Autodesk Inventor part; units mm, degrees
(part 2 of 2)
sketch "Sketch18" plane through (0, 0, -25.4) normal (0, 0, -1) x (-1, 0, 0)
  line L0 (16.4928, 228.3099) -> (15.5678, 226.2451) projected
  line L1 (15.5678, 226.2451) -> (12.4738, 226.4368) projected
  line L2 (12.4738, 226.4368) -> (11.8107, 228.5999) projected
  arc A0 (11.8107, 228.5999) -> (-2.4172, 228.892) centre (0, 0) ccw projected
  line L3 (-2.4172, 228.892) -> (-3.1685, 226.758) projected
  line L4 (-3.1685, 226.758) -> (-6.2678, 226.6935) projected
  line L5 (-6.2678, 226.6935) -> (-7.1073, 228.7944) projected
  arc A1 (-7.1073, 228.7944) -> (-11.8741, 228.5966) centre (0, 0) ccw projected
  line L6 (-11.8741, 228.5966) -> (-12.5366, 226.4333) projected
  line L7 (-12.5366, 226.4333) -> (-15.6306, 226.2408) projected
  line L8 (-15.6306, 226.2408) -> (-16.5561, 228.3053) projected
  arc A2 (-16.5561, 228.3053) -> (-21.3107, 227.9106) centre (0, 0) ccw projected
  line L9 (-21.3107, 227.9106) -> (-21.8832, 225.7218) projected
  line L10 (-21.8832, 225.7218) -> (-24.9666, 225.4016) projected
  line L11 (-24.9666, 225.4016) -> (-25.9767, 227.4261) projected
  arc A3 (-25.9767, 227.4261) -> (-30.7109, 226.8353) centre (0, 0) ccw projected
  line L12 (-30.7109, 226.8353) -> (-31.1925, 224.6247) projected
  line L13 (-31.1925, 224.6247) -> (-34.26, 224.1773) projected
  line L14 (-34.26, 224.1773) -> (-35.3529, 226.1583) projected
  arc A4 (-35.3529, 226.1583) -> (-40.0586, 225.3724) centre (0, 0) ccw projected
  line L15 (-40.0586, 225.3724) -> (-40.4484, 223.1438) projected
  line L16 (-40.4484, 223.1438) -> (-43.4949, 222.57) projected
  line L17 (-43.4949, 222.57) -> (-44.6687, 224.5042) projected
  arc A5 (-44.6687, 224.5042) -> (-49.3379, 223.5244) centre (0, 0) ccw projected
  line L18 (-49.3379, 223.5244) -> (-49.6353, 221.2816) projected
  line L19 (-49.6353, 221.2816) -> (-52.6554, 220.5825) projected
  line L20 (-52.6554, 220.5825) -> (-53.9082, 222.4664) projected
  arc A6 (-53.9082, 222.4664) -> (-58.5329, 221.2946) centre (0, 0) ccw projected
  line L21 (-58.5329, 221.2946) -> (-58.7374, 219.0414) projected
  line L22 (-58.7374, 219.0414) -> (-61.726, 218.218) projected
  line L23 (-61.726, 218.218) -> (-63.0555, 220.0486) projected
  arc A7 (-63.0555, 220.0486) -> (-67.6279, 218.6867) centre (0, 0) ccw projected
  line L24 (-67.6279, 218.6867) -> (-67.7391, 216.427) projected
  line L25 (-67.7391, 216.427) -> (-70.6911, 215.4808) projected
  line L26 (-70.6911, 215.4808) -> (-72.0952, 217.2549) projected
  arc A8 (-72.0952, 217.2549) -> (-76.6074, 215.7052) centre (0, 0) ccw projected
  line L27 (-76.6074, 215.7052) -> (-76.625, 213.4428) projected
  line L28 (-76.625, 213.4428) -> (-79.5355, 212.3754) projected
  line L29 (-79.5355, 212.3754) -> (-81.0116, 214.09) projected
  arc A9 (-81.0116, 214.09) -> (-85.4559, 212.3551) centre (0, 0) ccw projected
  line L30 (-85.4559, 212.3551) -> (-85.3801, 210.0939) projected
  line L31 (-85.3801, 210.0939) -> (-88.244, 208.9072) projected
  line L32 (-88.244, 208.9072) -> (-89.7897, 210.5593) projected
  arc A10 (-89.7897, 210.5593) -> (-94.1585, 208.6422) centre (0, 0) ccw projected
  line L33 (-94.1585, 208.6422) -> (-93.9893, 206.3861) projected
  line L34 (-93.9893, 206.3861) -> (-96.8017, 205.0821) projected
  line L35 (-96.8017, 205.0821) -> (-98.4143, 206.6689) projected
  arc A11 (-98.4143, 206.6689) -> (-102.7002, 204.5729) centre (0, 0) ccw projected
  line L36 (-102.7002, 204.5729) -> (-102.4379, 202.3257) projected
  line L37 (-102.4379, 202.3257) -> (-105.194, 200.9065) projected
  line L38 (-105.194, 200.9065) -> (-106.8709, 202.4254) projected
  arc A12 (-106.8709, 202.4254) -> (-111.0664, 200.1541) centre (0, 0) ccw projected
  line L39 (-111.0664, 200.1541) -> (-110.7115, 197.9196) projected
  line L40 (-110.7115, 197.9196) -> (-113.4066, 196.3878) projected
  line L41 (-113.4066, 196.3878) -> (-115.1448, 197.836) projected
  arc A13 (-115.1448, 197.836) -> (-119.2429, 195.3933) centre (0, 0) ccw projected
  line L42 (-119.2429, 195.3933) -> (-118.7959, 193.1754) projected
  line L43 (-118.7959, 193.1754) -> (-121.4254, 191.5335) projected
  line L44 (-121.4254, 191.5335) -> (-123.222, 192.9086) projected
  arc A14 (-123.222, 192.9086) -> (-127.2157, 190.2987) centre (0, 0) ccw projected
  line L45 (-127.2157, 190.2987) -> (-126.6774, 188.1011) projected
  line L46 (-126.6774, 188.1011) -> (-129.2368, 186.352) projected
  line L47 (-129.2368, 186.352) -> (-131.0887, 187.6517) projected
  arc A15 (-131.0887, 187.6517) -> (-134.9711, 184.8789) centre (0, 0) ccw projected
  line L48 (-134.9711, 184.8789) -> (-134.3425, 182.7055) projected
  line L49 (-134.3425, 182.7055) -> (-136.8274, 180.8521) projected
  line L50 (-136.8274, 180.8521) -> (-138.7314, 182.0742) projected
  arc A16 (-138.7314, 182.0742) -> (-142.4959, 179.1433) centre (0, 0) ccw projected
  line L51 (-142.4959, 179.1433) -> (-141.778, 176.9977) projected
  line L52 (-141.778, 176.9977) -> (-144.1842, 175.0432) projected
  line L53 (-144.1842, 175.0432) -> (-146.1371, 176.1856) projected
  arc A17 (-146.1371, 176.1856) -> (-149.7773, 173.1016) centre (0, 0) ccw projected
  line L54 (-149.7773, 173.1016) -> (-148.9713, 170.9876) projected
  line L55 (-148.9713, 170.9876) -> (-151.2947, 168.9353) projected
  line L56 (-151.2947, 168.9353) -> (-153.2931, 169.9959) projected
  arc A18 (-153.2931, 169.9959) -> (-156.8028, 166.7642) centre (0, 0) ccw projected
  line L57 (-156.8028, 166.7642) -> (-155.9101, 164.6853) projected
  line L58 (-155.9101, 164.6853) -> (-158.1467, 162.5387) projected
  line L59 (-158.1467, 162.5387) -> (-160.1873, 163.5159) projected
  arc A19 (-160.1873, 163.5159) -> (-163.5603, 160.1419) centre (0, 0) ccw projected
  line L60 (-163.5603, 160.1419) -> (-162.5826, 158.1016) projected
  line L61 (-162.5826, 158.1016) -> (-164.7285, 155.8644) projected
  line L62 (-164.7285, 155.8644) -> (-166.8077, 156.7565) projected
  arc A20 (-166.8077, 156.7565) -> (-170.0385, 153.246) centre (0, 0) ccw projected
  line L63 (-170.0385, 153.246) -> (-168.9772, 151.2478) projected
  line L64 (-168.9772, 151.2478) -> (-171.0289, 148.9239) projected
  line L65 (-171.0289, 148.9239) -> (-173.1432, 149.7292) projected
  arc A21 (-173.1432, 149.7292) -> (-176.2261, 146.0882) centre (0, 0) ccw projected
  line L66 (-176.2261, 146.0882) -> (-175.0832, 144.1357) projected
  line L67 (-175.0832, 144.1357) -> (-177.0371, 141.7289) projected
  line L68 (-177.0371, 141.7289) -> (-179.1828, 142.4462) projected
  arc A22 (-179.1828, 142.4462) -> (-182.1127, 138.6809) centre (0, 0) ccw projected
  line L69 (-182.1127, 138.6809) -> (-180.89, 136.7772) projected
  line L70 (-180.89, 136.7772) -> (-182.7428, 134.2918) projected
  line L71 (-182.7428, 134.2918) -> (-184.9163, 134.9198) projected
  arc A23 (-184.9163, 134.9198) -> (-187.6881, 131.0366) centre (0, 0) ccw projected
  line L72 (-187.6881, 131.0366) -> (-186.3878, 129.1851) projected
  line L73 (-186.3878, 129.1851) -> (-188.1363, 126.6252) projected
  line L74 (-188.1363, 126.6252) -> (-190.3339, 127.1629) projected
  arc A24 (-190.3339, 127.1629) -> (-192.9428, 123.1685) centre (0, 0) ccw projected
  line L75 (-192.9428, 123.1685) -> (-191.5672, 121.3723) projected
  line L76 (-191.5672, 121.3723) -> (-193.2084, 118.7423) projected
  line L77 (-193.2084, 118.7423) -> (-195.4264, 119.1887) projected
  arc A25 (-195.4264, 119.1887) -> (-197.8679, 115.0899) centre (0, 0) ccw projected
  line L78 (-197.8679, 115.0899) -> (-196.4192, 113.3521) projected
  line L79 (-196.4192, 113.3521) -> (-197.9503, 110.6566) projected
  line L80 (-197.9503, 110.6566) -> (-200.1849, 111.0109) projected
  arc A26 (-200.1849, 111.0109) -> (-202.455, 106.8147) centre (0, 0) ccw projected
  line L81 (-202.455, 106.8147) -> (-200.9357, 105.1382) projected
  line L82 (-200.9357, 105.1382) -> (-202.3541, 102.3818) projected
  line L83 (-202.3541, 102.3818) -> (-204.6014, 102.6434) projected
  arc A27 (-204.6014, 102.6434) -> (-206.6962, 98.357) centre (0, 0) ccw projected
  line L84 (-206.6962, 98.357) -> (-205.1089, 96.7448) projected
  line L85 (-205.1089, 96.7448) -> (-206.4122, 93.932) projected
  line L86 (-206.4122, 93.932) -> (-208.6684, 94.1006) projected
  arc A28 (-208.6684, 94.1006) -> (-210.5842, 89.7313) centre (0, 0) ccw projected
  line L87 (-210.5842, 89.7313) -> (-208.9317, 88.186) projected
  line L88 (-208.9317, 88.186) -> (-210.1176, 85.3218) projected
  line L89 (-210.1176, 85.3218) -> (-212.3788, 85.397) projected
  arc A29 (-212.3788, 85.397) -> (-214.1125, 80.9522) centre (0, 0) ccw projected
  line L90 (-214.1125, 80.9522) -> (-212.3975, 79.4766) projected
  line L91 (-212.3975, 79.4766) -> (-213.464, 76.5658) projected
  line L92 (-213.464, 76.5658) -> (-215.7264, 76.5475) projected
  arc A30 (-215.7264, 76.5475) -> (-217.2749, 72.0349) centre (0, 0) ccw projected
  line L93 (-217.2749, 72.0349) -> (-215.5004, 70.6313) projected
  line L94 (-215.5004, 70.6313) -> (-216.4458, 67.679) projected
  line L95 (-216.4458, 67.679) -> (-218.7055, 67.5672) projected
  arc A31 (-218.7055, 67.5672) -> (-220.0661, 62.9945) centre (0, 0) ccw projected
  line L96 (-220.0661, 62.9945) -> (-218.2352, 61.6655) projected
  line L97 (-218.2352, 61.6655) -> (-219.0577, 58.6766) projected
  line L98 (-219.0577, 58.6766) -> (-221.3108, 58.4715) projected
  arc A32 (-221.3108, 58.4715) -> (-222.4814, 53.8464) centre (0, 0) ccw projected
  line L99 (-222.4814, 53.8464) -> (-220.5971, 52.5942) projected
  line L100 (-220.5971, 52.5942) -> (-221.2954, 49.5739) projected
  line L101 (-221.2954, 49.5739) -> (-223.5381, 49.2759) projected
  arc A33 (-223.5381, 49.2759) -> (-224.5165, 44.6064) centre (0, 0) ccw projected
  line L102 (-224.5165, 44.6064) -> (-222.5821, 43.4331) projected
  line L103 (-222.5821, 43.4331) -> (-223.155, 40.3865) projected
  line L104 (-223.155, 40.3865) -> (-225.3835, 39.9961) projected
  arc A34 (-225.3835, 39.9961) -> (-226.1681, 35.2902) centre (0, 0) ccw projected
  line L105 (-226.1681, 35.2902) -> (-224.1868, 34.1978) projected
  line L106 (-224.1868, 34.1978) -> (-224.6333, 31.1302) projected
  line L107 (-224.6333, 31.1302) -> (-226.8438, 30.648) projected
  arc A35 (-226.8438, 30.648) -> (-227.4333, 25.9136) centre (0, 0) ccw projected
  line L108 (-227.4333, 25.9136) -> (-225.4085, 24.9041) projected
  line L109 (-225.4085, 24.9041) -> (-225.7279, 21.8206) projected
  line L110 (-225.7279, 21.8206) -> (-227.9165, 21.2475) projected
  arc A36 (-227.9165, 21.2475) -> (-228.3099, 16.4928) centre (0, 0) ccw projected
  line L111 (-228.3099, 16.4928) -> (-226.2451, 15.5678) projected
  line L112 (-226.2451, 15.5678) -> (-226.4368, 12.4738) projected
  line L113 (-226.4368, 12.4738) -> (-228.5999, 11.8107) projected
  arc A37 (-228.5999, 11.8107) -> (-228.7964, 7.0438) centre (0, 0) ccw projected
  line L114 (-228.7964, 7.0438) -> (-226.6952, 6.205) projected
  line L115 (-226.6952, 6.205) -> (-226.7588, 3.1056) projected
  line L116 (-226.7588, 3.1056) -> (-228.8927, 2.3537) projected
  arc A38 (-228.8927, 2.3537) -> (-228.892, -2.4172) centre (0, 0) ccw projected
  line L117 (-228.892, -2.4172) -> (-226.758, -3.1685) projected
  line L118 (-226.758, -3.1685) -> (-226.6935, -6.2678) projected
  line L119 (-226.6935, -6.2678) -> (-228.7944, -7.1073) projected
  arc A39 (-228.7944, -7.1073) -> (-228.5966, -11.8741) centre (0, 0) ccw projected
  line L120 (-228.5966, -11.8741) -> (-226.4333, -12.5366) projected
  line L121 (-226.4333, -12.5366) -> (-226.2408, -15.6306) projected
  line L122 (-226.2408, -15.6306) -> (-228.3053, -16.5561) projected
  arc A40 (-228.3053, -16.5561) -> (-227.9106, -21.3107) centre (0, 0) ccw projected
  line L123 (-227.9106, -21.3107) -> (-225.7218, -21.8832) projected
  line L124 (-225.7218, -21.8832) -> (-225.4016, -24.9666) projected
  line L125 (-225.4016, -24.9666) -> (-227.4261, -25.9767) projected
  arc A41 (-227.4261, -25.9767) -> (-226.8353, -30.7109) centre (0, 0) ccw projected
  line L126 (-226.8353, -30.7109) -> (-224.6247, -31.1925) projected
  line L127 (-224.6247, -31.1925) -> (-224.1773, -34.26) projected
  line L128 (-224.1773, -34.26) -> (-226.1583, -35.3529) projected
  arc A42 (-226.1583, -35.3529) -> (-225.3724, -40.0586) centre (0, 0) ccw projected
  line L129 (-225.3724, -40.0586) -> (-223.1438, -40.4484) projected
  line L130 (-223.1438, -40.4484) -> (-222.57, -43.4949) projected
  line L131 (-222.57, -43.4949) -> (-224.5042, -44.6687) projected
  arc A43 (-224.5042, -44.6687) -> (-223.5244, -49.3379) centre (0, 0) ccw projected
  line L132 (-223.5244, -49.3379) -> (-221.2816, -49.6353) projected
  line L133 (-221.2816, -49.6353) -> (-220.5825, -52.6554) projected
  line L134 (-220.5825, -52.6554) -> (-222.4664, -53.9082) projected
  arc A44 (-222.4664, -53.9082) -> (-221.2946, -58.5329) centre (0, 0) ccw projected
  line L135 (-221.2946, -58.5329) -> (-219.0414, -58.7374) projected
  line L136 (-219.0414, -58.7374) -> (-218.218, -61.726) projected
  line L137 (-218.218, -61.726) -> (-220.0486, -63.0555) projected
  arc A45 (-220.0486, -63.0555) -> (-218.6867, -67.6279) centre (0, 0) ccw projected
  line L138 (-218.6867, -67.6279) -> (-216.427, -67.7391) projected
  line L139 (-216.427, -67.7391) -> (-215.4808, -70.6911) projected
  line L140 (-215.4808, -70.6911) -> (-217.2549, -72.0952) projected
  arc A46 (-217.2549, -72.0952) -> (-215.7052, -76.6074) centre (0, 0) ccw projected
  line L141 (-215.7052, -76.6074) -> (-213.4428, -76.625) projected
  line L142 (-213.4428, -76.625) -> (-212.3754, -79.5355) projected
  line L143 (-212.3754, -79.5355) -> (-214.09, -81.0116) projected
  arc A47 (-214.09, -81.0116) -> (-212.3551, -85.4559) centre (0, 0) ccw projected
  line L144 (-212.3551, -85.4559) -> (-210.0939, -85.3801) projected
  line L145 (-210.0939, -85.3801) -> (-208.9072, -88.244) projected
  line L146 (-208.9072, -88.244) -> (-210.5593, -89.7897) projected
  arc A48 (-210.5593, -89.7897) -> (-208.6422, -94.1585) centre (0, 0) ccw projected
  line L147 (-208.6422, -94.1585) -> (-206.3861, -93.9893) projected
  line L148 (-206.3861, -93.9893) -> (-205.0821, -96.8017) projected
  line L149 (-205.0821, -96.8017) -> (-206.6689, -98.4143) projected
  arc A49 (-206.6689, -98.4143) -> (-204.5729, -102.7002) centre (0, 0) ccw projected
  line L150 (-204.5729, -102.7002) -> (-202.3257, -102.4379) projected
  line L151 (-202.3257, -102.4379) -> (-200.9065, -105.194) projected
  line L152 (-200.9065, -105.194) -> (-202.4254, -106.8709) projected
  arc A50 (-202.4254, -106.8709) -> (-200.1541, -111.0664) centre (0, 0) ccw projected
  line L153 (-200.1541, -111.0664) -> (-197.9196, -110.7115) projected
  line L154 (-197.9196, -110.7115) -> (-196.3878, -113.4066) projected
  line L155 (-196.3878, -113.4066) -> (-197.836, -115.1448) projected
  arc A51 (-197.836, -115.1448) -> (-195.3933, -119.2429) centre (0, 0) ccw projected
  line L156 (-195.3933, -119.2429) -> (-193.1754, -118.7959) projected
  line L157 (-193.1754, -118.7959) -> (-191.5335, -121.4254) projected
  line L158 (-191.5335, -121.4254) -> (-192.9086, -123.222) projected
  arc A52 (-192.9086, -123.222) -> (-190.2987, -127.2157) centre (0, 0) ccw projected
  line L159 (-190.2987, -127.2157) -> (-188.1011, -126.6774) projected
  line L160 (-188.1011, -126.6774) -> (-186.352, -129.2368) projected
  line L161 (-186.352, -129.2368) -> (-187.6517, -131.0887) projected
  arc A53 (-187.6517, -131.0887) -> (-184.8789, -134.9711) centre (0, 0) ccw projected
  line L162 (-184.8789, -134.9711) -> (-182.7055, -134.3425) projected
  line L163 (-182.7055, -134.3425) -> (-180.8521, -136.8274) projected
  line L164 (-180.8521, -136.8274) -> (-182.0742, -138.7314) projected
  arc A54 (-182.0742, -138.7314) -> (-179.1433, -142.4959) centre (0, 0) ccw projected
  line L165 (-179.1433, -142.4959) -> (-176.9977, -141.778) projected
  line L166 (-176.9977, -141.778) -> (-175.0432, -144.1842) projected
  line L167 (-175.0432, -144.1842) -> (-176.1856, -146.1371) projected
  arc A55 (-176.1856, -146.1371) -> (-173.1016, -149.7773) centre (0, 0) ccw projected
  line L168 (-173.1016, -149.7773) -> (-170.9876, -148.9713) projected
  line L169 (-170.9876, -148.9713) -> (-168.9353, -151.2947) projected
  line L170 (-168.9353, -151.2947) -> (-169.9959, -153.2931) projected
  arc A56 (-169.9959, -153.2931) -> (-166.7642, -156.8028) centre (0, 0) ccw projected
  line L171 (-166.7642, -156.8028) -> (-164.6853, -155.9101) projected
  line L172 (-164.6853, -155.9101) -> (-162.5387, -158.1467) projected
  line L173 (-162.5387, -158.1467) -> (-163.5159, -160.1873) projected
  arc A57 (-163.5159, -160.1873) -> (-160.1419, -163.5603) centre (0, 0) ccw projected
  line L174 (-160.1419, -163.5603) -> (-158.1016, -162.5826) projected
  line L175 (-158.1016, -162.5826) -> (-155.8644, -164.7285) projected
  line L176 (-155.8644, -164.7285) -> (-156.7565, -166.8077) projected
  arc A58 (-156.7565, -166.8077) -> (-153.246, -170.0385) centre (0, 0) ccw projected
  line L177 (-153.246, -170.0385) -> (-151.2478, -168.9772) projected
  line L178 (-151.2478, -168.9772) -> (-148.9239, -171.0289) projected
  line L179 (-148.9239, -171.0289) -> (-149.7292, -173.1432) projected
  arc A59 (-149.7292, -173.1432) -> (-146.0882, -176.2261) centre (0, 0) ccw projected
  line L180 (-146.0882, -176.2261) -> (-144.1357, -175.0832) projected
  line L181 (-144.1357, -175.0832) -> (-141.7289, -177.0371) projected
  line L182 (-141.7289, -177.0371) -> (-142.4462, -179.1828) projected
  arc A60 (-142.4462, -179.1828) -> (-138.6809, -182.1127) centre (0, 0) ccw projected
  line L183 (-138.6809, -182.1127) -> (-136.7772, -180.89) projected
  line L184 (-136.7772, -180.89) -> (-134.2918, -182.7428) projected
  line L185 (-134.2918, -182.7428) -> (-134.9198, -184.9163) projected
  arc A61 (-134.9198, -184.9163) -> (-131.0366, -187.6881) centre (0, 0) ccw projected
  line L186 (-131.0366, -187.6881) -> (-129.1851, -186.3878) projected
  line L187 (-129.1851, -186.3878) -> (-126.6252, -188.1363) projected
  line L188 (-126.6252, -188.1363) -> (-127.1629, -190.3339) projected
  arc A62 (-127.1629, -190.3339) -> (-123.1685, -192.9428) centre (0, 0) ccw projected
  line L189 (-123.1685, -192.9428) -> (-121.3723, -191.5672) projected
  line L190 (-121.3723, -191.5672) -> (-118.7423, -193.2084) projected
  line L191 (-118.7423, -193.2084) -> (-119.1887, -195.4264) projected
  arc A63 (-119.1887, -195.4264) -> (-115.0899, -197.8679) centre (0, 0) ccw projected
  line L192 (-115.0899, -197.8679) -> (-113.3521, -196.4192) projected
  line L193 (-113.3521, -196.4192) -> (-110.6566, -197.9503) projected
  line L194 (-110.6566, -197.9503) -> (-111.0109, -200.1849) projected
  arc A64 (-111.0109, -200.1849) -> (-106.8147, -202.455) centre (0, 0) ccw projected
  line L195 (-106.8147, -202.455) -> (-105.1382, -200.9357) projected
  line L196 (-105.1382, -200.9357) -> (-102.3818, -202.3541) projected
  line L197 (-102.3818, -202.3541) -> (-102.6434, -204.6014) projected
  arc A65 (-102.6434, -204.6014) -> (-98.357, -206.6962) centre (0, 0) ccw projected
  line L198 (-98.357, -206.6962) -> (-96.7448, -205.1089) projected
  line L199 (-96.7448, -205.1089) -> (-93.932, -206.4122) projected
  line L200 (-93.932, -206.4122) -> (-94.1006, -208.6684) projected
  arc A66 (-94.1006, -208.6684) -> (-89.7313, -210.5842) centre (0, 0) ccw projected
  line L201 (-89.7313, -210.5842) -> (-88.186, -208.9317) projected
  line L202 (-88.186, -208.9317) -> (-85.3218, -210.1176) projected
  line L203 (-85.3218, -210.1176) -> (-85.397, -212.3788) projected
  arc A67 (-85.397, -212.3788) -> (-80.9522, -214.1125) centre (0, 0) ccw projected
  line L204 (-80.9522, -214.1125) -> (-79.4766, -212.3975) projected
  line L205 (-79.4766, -212.3975) -> (-76.5658, -213.464) projected
  line L206 (-76.5658, -213.464) -> (-76.5475, -215.7264) projected
  arc A68 (-76.5475, -215.7264) -> (-72.0349, -217.2749) centre (0, 0) ccw projected
  line L207 (-72.0349, -217.2749) -> (-70.6313, -215.5004) projected
  line L208 (-70.6313, -215.5004) -> (-67.679, -216.4458) projected
  line L209 (-67.679, -216.4458) -> (-67.5672, -218.7055) projected
  arc A69 (-67.5672, -218.7055) -> (-62.9945, -220.0661) centre (0, 0) ccw projected
  line L210 (-62.9945, -220.0661) -> (-61.6655, -218.2352) projected
  line L211 (-61.6655, -218.2352) -> (-58.6766, -219.0577) projected
  line L212 (-58.6766, -219.0577) -> (-58.4715, -221.3108) projected
  arc A70 (-58.4715, -221.3108) -> (-53.8464, -222.4814) centre (0, 0) ccw projected
  line L213 (-53.8464, -222.4814) -> (-52.5942, -220.5971) projected
  line L214 (-52.5942, -220.5971) -> (-49.5739, -221.2954) projected
  line L215 (-49.5739, -221.2954) -> (-49.2759, -223.5381) projected
  arc A71 (-49.2759, -223.5381) -> (-44.6064, -224.5165) centre (0, 0) ccw projected
  line L216 (-44.6064, -224.5165) -> (-43.4331, -222.5821) projected
  line L217 (-43.4331, -222.5821) -> (-40.3865, -223.155) projected
  line L218 (-40.3865, -223.155) -> (-39.9961, -225.3835) projected
  arc A72 (-39.9961, -225.3835) -> (-35.2902, -226.1681) centre (0, 0) ccw projected
  line L219 (-35.2902, -226.1681) -> (-34.1978, -224.1868) projected
  line L220 (-34.1978, -224.1868) -> (-31.1302, -224.6333) projected
  line L221 (-31.1302, -224.6333) -> (-30.648, -226.8438) projected
  arc A73 (-30.648, -226.8438) -> (-25.9136, -227.4333) centre (0, 0) ccw projected
  line L222 (-25.9136, -227.4333) -> (-24.9041, -225.4085) projected
  line L223 (-24.9041, -225.4085) -> (-21.8206, -225.7279) projected
  line L224 (-21.8206, -225.7279) -> (-21.2475, -227.9165) projected
  arc A74 (-21.2475, -227.9165) -> (-16.4928, -228.3099) centre (0, 0) ccw projected
  line L225 (-16.4928, -228.3099) -> (-15.5678, -226.2451) projected
  line L226 (-15.5678, -226.2451) -> (-12.4738, -226.4368) projected
  line L227 (-12.4738, -226.4368) -> (-11.8107, -228.5999) projected
  arc A75 (-11.8107, -228.5999) -> (-7.0438, -228.7964) centre (0, 0) ccw projected
  line L228 (-7.0438, -228.7964) -> (-6.205, -226.6952) projected
  line L229 (-6.205, -226.6952) -> (-3.1056, -226.7588) projected
  line L230 (-3.1056, -226.7588) -> (-2.3537, -228.8927) projected
  arc A76 (-2.3537, -228.8927) -> (2.4172, -228.892) centre (0, 0) ccw projected
  line L231 (2.4172, -228.892) -> (3.1685, -226.758) projected
  line L232 (3.1685, -226.758) -> (6.2678, -226.6935) projected
  line L233 (6.2678, -226.6935) -> (7.1073, -228.7944) projected
  arc A77 (7.1073, -228.7944) -> (11.8741, -228.5966) centre (0, 0) ccw projected
  line L234 (11.8741, -228.5966) -> (12.5366, -226.4333) projected
  line L235 (12.5366, -226.4333) -> (15.6306, -226.2408) projected
  line L236 (15.6306, -226.2408) -> (16.5561, -228.3053) projected
  arc A78 (16.5561, -228.3053) -> (21.3107, -227.9106) centre (0, 0) ccw projected
  line L237 (21.3107, -227.9106) -> (21.8832, -225.7218) projected
  line L238 (21.8832, -225.7218) -> (24.9666, -225.4016) projected
  line L239 (24.9666, -225.4016) -> (25.9767, -227.4261) projected
  arc A79 (25.9767, -227.4261) -> (30.7109, -226.8353) centre (0, 0) ccw projected
  line L240 (30.7109, -226.8353) -> (31.1925, -224.6247) projected
  line L241 (31.1925, -224.6247) -> (34.26, -224.1773) projected
  line L242 (34.26, -224.1773) -> (35.3529, -226.1583) projected
  arc A80 (35.3529, -226.1583) -> (40.0586, -225.3724) centre (0, 0) ccw projected
  line L243 (40.0586, -225.3724) -> (40.4484, -223.1438) projected
  line L244 (40.4484, -223.1438) -> (43.4949, -222.57) projected
  line L245 (43.4949, -222.57) -> (44.6687, -224.5042) projected
  arc A81 (44.6687, -224.5042) -> (49.3379, -223.5244) centre (0, 0) ccw projected
  line L246 (49.3379, -223.5244) -> (49.6353, -221.2816) projected
  line L247 (49.6353, -221.2816) -> (52.6554, -220.5825) projected
  line L248 (52.6554, -220.5825) -> (53.9082, -222.4664) projected
  arc A82 (53.9082, -222.4664) -> (58.5329, -221.2946) centre (0, 0) ccw projected
  line L249 (58.5329, -221.2946) -> (58.7374, -219.0414) projected
  line L250 (58.7374, -219.0414) -> (61.726, -218.218) projected
  line L251 (61.726, -218.218) -> (63.0555, -220.0486) projected
  arc A83 (63.0555, -220.0486) -> (67.6279, -218.6867) centre (0, 0) ccw projected
  line L252 (67.6279, -218.6867) -> (67.7391, -216.427) projected
  line L253 (67.7391, -216.427) -> (70.6911, -215.4808) projected
  line L254 (70.6911, -215.4808) -> (72.0952, -217.2549) projected
  arc A84 (72.0952, -217.2549) -> (76.6074, -215.7052) centre (0, 0) ccw projected
  line L255 (76.6074, -215.7052) -> (76.625, -213.4428) projected
  line L256 (76.625, -213.4428) -> (79.5355, -212.3754) projected
  line L257 (79.5355, -212.3754) -> (81.0116, -214.09) projected
  arc A85 (81.0116, -214.09) -> (85.4559, -212.3551) centre (0, 0) ccw projected
  line L258 (85.4559, -212.3551) -> (85.3801, -210.0939) projected
  line L259 (85.3801, -210.0939) -> (88.244, -208.9072) projected
  line L260 (88.244, -208.9072) -> (89.7897, -210.5593) projected
  arc A86 (89.7897, -210.5593) -> (94.1585, -208.6422) centre (0, 0) ccw projected
  line L261 (94.1585, -208.6422) -> (93.9893, -206.3861) projected
  line L262 (93.9893, -206.3861) -> (96.8017, -205.0821) projected
  line L263 (96.8017, -205.0821) -> (98.4143, -206.6689) projected
  arc A87 (98.4143, -206.6689) -> (102.7002, -204.5729) centre (0, 0) ccw projected
  line L264 (102.7002, -204.5729) -> (102.4379, -202.3257) projected
  line L265 (102.4379, -202.3257) -> (105.194, -200.9065) projected
  line L266 (105.194, -200.9065) -> (106.8709, -202.4254) projected
  arc A88 (106.8709, -202.4254) -> (111.0664, -200.1541) centre (0, 0) ccw projected
  line L267 (111.0664, -200.1541) -> (110.7115, -197.9196) projected
  line L268 (110.7115, -197.9196) -> (113.4066, -196.3878) projected
  line L269 (113.4066, -196.3878) -> (115.1448, -197.836) projected
  arc A89 (115.1448, -197.836) -> (119.2429, -195.3933) centre (0, 0) ccw projected
  line L270 (119.2429, -195.3933) -> (118.7959, -193.1754) projected
  line L271 (118.7959, -193.1754) -> (121.4254, -191.5335) projected
  line L272 (121.4254, -191.5335) -> (123.222, -192.9086) projected
  arc A90 (123.222, -192.9086) -> (127.2157, -190.2987) centre (0, 0) ccw projected
  line L273 (127.2157, -190.2987) -> (126.6774, -188.1011) projected
  line L274 (126.6774, -188.1011) -> (129.2368, -186.352) projected
  line L275 (129.2368, -186.352) -> (131.0887, -187.6517) projected
  arc A91 (131.0887, -187.6517) -> (134.9711, -184.8789) centre (0, 0) ccw projected
  line L276 (134.9711, -184.8789) -> (134.3425, -182.7055) projected
  line L277 (134.3425, -182.7055) -> (136.8274, -180.8521) projected
  line L278 (136.8274, -180.8521) -> (138.7314, -182.0742) projected
  arc A92 (138.7314, -182.0742) -> (142.4959, -179.1433) centre (0, 0) ccw projected
  line L279 (142.4959, -179.1433) -> (141.778, -176.9977) projected
  line L280 (141.778, -176.9977) -> (144.1842, -175.0432) projected
  line L281 (144.1842, -175.0432) -> (146.1371, -176.1856) projected
  arc A93 (146.1371, -176.1856) -> (149.7773, -173.1016) centre (0, 0) ccw projected
  line L282 (149.7773, -173.1016) -> (148.9713, -170.9876) projected
  line L283 (148.9713, -170.9876) -> (151.2947, -168.9353) projected
  line L284 (151.2947, -168.9353) -> (153.2931, -169.9959) projected
  arc A94 (153.2931, -169.9959) -> (156.8028, -166.7642) centre (0, 0) ccw projected
  line L285 (156.8028, -166.7642) -> (155.9101, -164.6853) projected
  line L286 (155.9101, -164.6853) -> (158.1467, -162.5387) projected
  line L287 (158.1467, -162.5387) -> (160.1873, -163.5159) projected
  arc A95 (160.1873, -163.5159) -> (163.5603, -160.1419) centre (0, 0) ccw projected
  line L288 (163.5603, -160.1419) -> (162.5826, -158.1016) projected
  line L289 (162.5826, -158.1016) -> (164.7285, -155.8644) projected
  line L290 (164.7285, -155.8644) -> (166.8077, -156.7565) projected
  arc A96 (166.8077, -156.7565) -> (170.0385, -153.246) centre (0, 0) ccw projected
  line L291 (170.0385, -153.246) -> (168.9772, -151.2478) projected
  line L292 (168.9772, -151.2478) -> (171.0289, -148.9239) projected
  line L293 (171.0289, -148.9239) -> (173.1432, -149.7292) projected
  arc A97 (173.1432, -149.7292) -> (176.2261, -146.0882) centre (0, 0) ccw projected
  line L294 (176.2261, -146.0882) -> (175.0832, -144.1357) projected
  line L295 (175.0832, -144.1357) -> (177.0371, -141.7289) projected
  line L296 (177.0371, -141.7289) -> (179.1828, -142.4462) projected
  arc A98 (179.1828, -142.4462) -> (182.1127, -138.6809) centre (0, 0) ccw projected
  line L297 (182.1127, -138.6809) -> (180.89, -136.7772) projected
  line L298 (180.89, -136.7772) -> (182.7428, -134.2918) projected
  line L299 (182.7428, -134.2918) -> (184.9163, -134.9198) projected
  arc A99 (184.9163, -134.9198) -> (187.6881, -131.0366) centre (0, 0) ccw projected
  line L300 (187.6881, -131.0366) -> (186.3878, -129.1851) projected
  line L301 (186.3878, -129.1851) -> (188.1363, -126.6252) projected
  line L302 (188.1363, -126.6252) -> (190.3339, -127.1629) projected
  arc A100 (190.3339, -127.1629) -> (192.9428, -123.1685) centre (0, 0) ccw projected
  line L303 (192.9428, -123.1685) -> (191.5672, -121.3723) projected
  line L304 (191.5672, -121.3723) -> (193.2084, -118.7423) projected
  line L305 (193.2084, -118.7423) -> (195.4264, -119.1887) projected
  arc A101 (195.4264, -119.1887) -> (197.8679, -115.0899) centre (0, 0) ccw projected
  line L306 (197.8679, -115.0899) -> (196.4192, -113.3521) projected
  line L307 (196.4192, -113.3521) -> (197.9503, -110.6566) projected
  line L308 (197.9503, -110.6566) -> (200.1849, -111.0109) projected
  arc A102 (200.1849, -111.0109) -> (202.455, -106.8147) centre (0, 0) ccw projected
  line L309 (202.455, -106.8147) -> (200.9357, -105.1382) projected
  line L310 (200.9357, -105.1382) -> (202.3541, -102.3818) projected
  line L311 (202.3541, -102.3818) -> (204.6014, -102.6434) projected
  arc A103 (204.6014, -102.6434) -> (206.6962, -98.357) centre (0, 0) ccw projected
  line L312 (206.6962, -98.357) -> (205.1089, -96.7448) projected
  line L313 (205.1089, -96.7448) -> (206.4122, -93.932) projected
  line L314 (206.4122, -93.932) -> (208.6684, -94.1006) projected
  arc A104 (208.6684, -94.1006) -> (210.5842, -89.7313) centre (0, 0) ccw projected
  line L315 (210.5842, -89.7313) -> (208.9317, -88.186) projected
  line L316 (208.9317, -88.186) -> (210.1176, -85.3218) projected
  line L317 (210.1176, -85.3218) -> (212.3788, -85.397) projected
  arc A105 (212.3788, -85.397) -> (214.1125, -80.9522) centre (0, 0) ccw projected
  line L318 (214.1125, -80.9522) -> (212.3975, -79.4766) projected
  line L319 (212.3975, -79.4766) -> (213.464, -76.5658) projected
  line L320 (213.464, -76.5658) -> (215.7264, -76.5475) projected
  arc A106 (215.7264, -76.5475) -> (217.2749, -72.0349) centre (0, 0) ccw projected
  line L321 (217.2749, -72.0349) -> (215.5004, -70.6313) projected
  line L322 (215.5004, -70.6313) -> (216.4458, -67.679) projected
  line L323 (216.4458, -67.679) -> (218.7055, -67.5672) projected
  arc A107 (218.7055, -67.5672) -> (220.0661, -62.9945) centre (0, 0) ccw projected
  line L324 (220.0661, -62.9945) -> (218.2352, -61.6655) projected
  line L325 (218.2352, -61.6655) -> (219.0577, -58.6766) projected
  line L326 (219.0577, -58.6766) -> (221.3108, -58.4715) projected
  arc A108 (221.3108, -58.4715) -> (222.4814, -53.8464) centre (0, 0) ccw projected
  line L327 (222.4814, -53.8464) -> (220.5971, -52.5942) projected
  line L328 (220.5971, -52.5942) -> (221.2954, -49.5739) projected
  line L329 (221.2954, -49.5739) -> (223.5381, -49.2759) projected
  arc A109 (223.5381, -49.2759) -> (224.5165, -44.6064) centre (0, 0) ccw projected
  line L330 (224.5165, -44.6064) -> (222.5821, -43.4331) projected
  line L331 (222.5821, -43.4331) -> (223.155, -40.3865) projected
  line L332 (223.155, -40.3865) -> (225.3835, -39.9961) projected
  arc A110 (225.3835, -39.9961) -> (226.1681, -35.2902) centre (0, 0) ccw projected
  line L333 (226.1681, -35.2902) -> (224.1868, -34.1978) projected
  line L334 (224.1868, -34.1978) -> (224.6333, -31.1302) projected
  line L335 (224.6333, -31.1302) -> (226.8438, -30.648) projected
  arc A111 (226.8438, -30.648) -> (227.4333, -25.9136) centre (0, 0) ccw projected
  line L336 (227.4333, -25.9136) -> (225.4085, -24.9041) projected
  line L337 (225.4085, -24.9041) -> (225.7279, -21.8206) projected
  line L338 (225.7279, -21.8206) -> (227.9165, -21.2475) projected
  arc A112 (227.9165, -21.2475) -> (228.3099, -16.4928) centre (0, 0) ccw projected
  line L339 (228.3099, -16.4928) -> (226.2451, -15.5678) projected
  line L340 (226.2451, -15.5678) -> (226.4368, -12.4738) projected
  line L341 (226.4368, -12.4738) -> (228.5999, -11.8107) projected
  arc A113 (228.5999, -11.8107) -> (228.7964, -7.0438) centre (0, 0) ccw projected
  line L342 (228.7964, -7.0438) -> (226.6952, -6.205) projected
  line L343 (226.6952, -6.205) -> (226.7588, -3.1056) projected
  line L344 (226.7588, -3.1056) -> (228.8927, -2.3537) projected
  arc A114 (228.8927, -2.3537) -> (228.892, 2.4172) centre (0, 0) ccw projected
  line L345 (228.892, 2.4172) -> (226.758, 3.1685) projected
  line L346 (226.758, 3.1685) -> (226.6935, 6.2678) projected
  line L347 (226.6935, 6.2678) -> (228.7944, 7.1073) projected
  arc A115 (228.7944, 7.1073) -> (228.5966, 11.8741) centre (0, 0) ccw projected
  line L348 (228.5966, 11.8741) -> (226.4333, 12.5366) projected
  line L349 (226.4333, 12.5366) -> (226.2408, 15.6306) projected
  line L350 (226.2408, 15.6306) -> (228.3053, 16.5561) projected
  arc A116 (228.3053, 16.5561) -> (227.9106, 21.3107) centre (0, 0) ccw projected
  line L351 (227.9106, 21.3107) -> (225.7218, 21.8832) projected
  line L352 (225.7218, 21.8832) -> (225.4016, 24.9666) projected
  line L353 (225.4016, 24.9666) -> (227.4261, 25.9767) projected
  arc A117 (227.4261, 25.9767) -> (226.8353, 30.7109) centre (0, 0) ccw projected
  line L354 (226.8353, 30.7109) -> (224.6247, 31.1925) projected
  line L355 (224.6247, 31.1925) -> (224.1773, 34.26) projected
  line L356 (224.1773, 34.26) -> (226.1583, 35.3529) projected
  arc A118 (226.1583, 35.3529) -> (225.3724, 40.0586) centre (0, 0) ccw projected
  line L357 (225.3724, 40.0586) -> (223.1438, 40.4484) projected
  line L358 (223.1438, 40.4484) -> (222.57, 43.4949) projected
  line L359 (222.57, 43.4949) -> (224.5042, 44.6687) projected
  arc A119 (224.5042, 44.6687) -> (223.5244, 49.3379) centre (0, 0) ccw projected
  line L360 (223.5244, 49.3379) -> (221.2816, 49.6353) projected
  line L361 (221.2816, 49.6353) -> (220.5825, 52.6554) projected
  line L362 (220.5825, 52.6554) -> (222.4664, 53.9082) projected
  arc A120 (222.4664, 53.9082) -> (221.2946, 58.5329) centre (0, 0) ccw projected
  line L363 (221.2946, 58.5329) -> (219.0414, 58.7374) projected
  line L364 (219.0414, 58.7374) -> (218.218, 61.726) projected
  line L365 (218.218, 61.726) -> (220.0486, 63.0555) projected
  arc A121 (220.0486, 63.0555) -> (218.6867, 67.6279) centre (0, 0) ccw projected
  line L366 (218.6867, 67.6279) -> (216.427, 67.7391) projected
  line L367 (216.427, 67.7391) -> (215.4808, 70.6911) projected
  line L368 (215.4808, 70.6911) -> (217.2549, 72.0952) projected
  arc A122 (217.2549, 72.0952) -> (215.7052, 76.6074) centre (0, 0) ccw projected
  line L369 (215.7052, 76.6074) -> (213.4428, 76.625) projected
  line L370 (213.4428, 76.625) -> (212.3754, 79.5355) projected
  line L371 (212.3754, 79.5355) -> (214.09, 81.0116) projected
  arc A123 (214.09, 81.0116) -> (212.3551, 85.4559) centre (0, 0) ccw projected
  line L372 (212.3551, 85.4559) -> (210.0939, 85.3801) projected
  line L373 (210.0939, 85.3801) -> (208.9072, 88.244) projected
  line L374 (208.9072, 88.244) -> (210.5593, 89.7897) projected
  arc A124 (210.5593, 89.7897) -> (208.6422, 94.1585) centre (0, 0) ccw projected
  line L375 (208.6422, 94.1585) -> (206.3861, 93.9893) projected
  line L376 (206.3861, 93.9893) -> (205.0821, 96.8017) projected
  line L377 (205.0821, 96.8017) -> (206.6689, 98.4143) projected
  arc A125 (206.6689, 98.4143) -> (204.5729, 102.7002) centre (0, 0) ccw projected
  line L378 (204.5729, 102.7002) -> (202.3257, 102.4379) projected
  line L379 (202.3257, 102.4379) -> (200.9065, 105.194) projected
  line L380 (200.9065, 105.194) -> (202.4254, 106.8709) projected
  arc A126 (202.4254, 106.8709) -> (200.1541, 111.0664) centre (0, 0) ccw projected
  line L381 (200.1541, 111.0664) -> (197.9196, 110.7115) projected
  line L382 (197.9196, 110.7115) -> (196.3878, 113.4066) projected
  line L383 (196.3878, 113.4066) -> (197.836, 115.1448) projected
  arc A127 (197.836, 115.1448) -> (195.3933, 119.2429) centre (0, 0) ccw projected
  line L384 (195.3933, 119.2429) -> (193.1754, 118.7959) projected
  line L385 (193.1754, 118.7959) -> (191.5335, 121.4254) projected
  line L386 (191.5335, 121.4254) -> (192.9086, 123.222) projected
  arc A128 (192.9086, 123.222) -> (190.2987, 127.2157) centre (0, 0) ccw projected
  line L387 (190.2987, 127.2157) -> (188.1011, 126.6774) projected
  line L388 (188.1011, 126.6774) -> (186.352, 129.2368) projected
  line L389 (186.352, 129.2368) -> (187.6517, 131.0887) projected
  arc A129 (187.6517, 131.0887) -> (184.8789, 134.9711) centre (0, 0) ccw projected
  line L390 (184.8789, 134.9711) -> (182.7055, 134.3425) projected
  line L391 (182.7055, 134.3425) -> (180.8521, 136.8274) projected
  line L392 (180.8521, 136.8274) -> (182.0742, 138.7314) projected
  arc A130 (182.0742, 138.7314) -> (179.1433, 142.4959) centre (0, 0) ccw projected
  line L393 (179.1433, 142.4959) -> (176.9977, 141.778) projected
  line L394 (176.9977, 141.778) -> (175.0432, 144.1842) projected
  line L395 (175.0432, 144.1842) -> (176.1856, 146.1371) projected
  arc A131 (176.1856, 146.1371) -> (173.1016, 149.7773) centre (0, 0) ccw projected
  line L396 (173.1016, 149.7773) -> (170.9876, 148.9713) projected
  line L397 (170.9876, 148.9713) -> (168.9353, 151.2947) projected
  line L398 (168.9353, 151.2947) -> (169.9959, 153.2931) projected
  arc A132 (169.9959, 153.2931) -> (166.7642, 156.8028) centre (0, 0) ccw projected
  line L399 (166.7642, 156.8028) -> (164.6853, 155.9101) projected
  line L400 (164.6853, 155.9101) -> (162.5387, 158.1467) projected
  line L401 (162.5387, 158.1467) -> (163.5159, 160.1873) projected
  arc A133 (163.5159, 160.1873) -> (160.1419, 163.5603) centre (0, 0) ccw projected
  line L402 (160.1419, 163.5603) -> (158.1016, 162.5826) projected
  line L403 (158.1016, 162.5826) -> (155.8644, 164.7285) projected
  line L404 (155.8644, 164.7285) -> (156.7565, 166.8077) projected
  arc A134 (156.7565, 166.8077) -> (153.246, 170.0385) centre (0, 0) ccw projected
  line L405 (153.246, 170.0385) -> (151.2478, 168.9772) projected
  line L406 (151.2478, 168.9772) -> (148.9239, 171.0289) projected
  line L407 (148.9239, 171.0289) -> (149.7292, 173.1432) projected
  arc A135 (149.7292, 173.1432) -> (146.0882, 176.2261) centre (0, 0) ccw projected
  line L408 (146.0882, 176.2261) -> (144.1357, 175.0832) projected
  line L409 (144.1357, 175.0832) -> (141.7289, 177.0371) projected
  line L410 (141.7289, 177.0371) -> (142.4462, 179.1828) projected
  arc A136 (142.4462, 179.1828) -> (138.6809, 182.1127) centre (0, 0) ccw projected
  line L411 (138.6809, 182.1127) -> (136.7772, 180.89) projected
  line L412 (136.7772, 180.89) -> (134.2918, 182.7428) projected
  line L413 (134.2918, 182.7428) -> (134.9198, 184.9163) projected
  arc A137 (134.9198, 184.9163) -> (131.0366, 187.6881) centre (0, 0) ccw projected
  line L414 (131.0366, 187.6881) -> (129.1851, 186.3878) projected
  line L415 (129.1851, 186.3878) -> (126.6252, 188.1363) projected
  line L416 (126.6252, 188.1363) -> (127.1629, 190.3339) projected
  arc A138 (127.1629, 190.3339) -> (123.1685, 192.9428) centre (0, 0) ccw projected
  line L417 (123.1685, 192.9428) -> (121.3723, 191.5672) projected
  line L418 (121.3723, 191.5672) -> (118.7423, 193.2084) projected
  line L419 (118.7423, 193.2084) -> (119.1887, 195.4264) projected
  arc A139 (119.1887, 195.4264) -> (115.0899, 197.8679) centre (0, 0) ccw projected
  line L420 (115.0899, 197.8679) -> (113.3521, 196.4192) projected
  line L421 (113.3521, 196.4192) -> (110.6566, 197.9503) projected
  line L422 (110.6566, 197.9503) -> (111.0109, 200.1849) projected
  arc A140 (111.0109, 200.1849) -> (106.8147, 202.455) centre (0, 0) ccw projected
  line L423 (106.8147, 202.455) -> (105.1382, 200.9357) projected
  line L424 (105.1382, 200.9357) -> (102.3818, 202.3541) projected
  line L425 (102.3818, 202.3541) -> (102.6434, 204.6014) projected
  arc A141 (102.6434, 204.6014) -> (98.357, 206.6962) centre (0, 0) ccw projected
  line L426 (98.357, 206.6962) -> (96.7448, 205.1089) projected
  line L427 (96.7448, 205.1089) -> (93.932, 206.4122) projected
  line L428 (93.932, 206.4122) -> (94.1006, 208.6684) projected
  arc A142 (94.1006, 208.6684) -> (89.7313, 210.5842) centre (0, 0) ccw projected
  line L429 (89.7313, 210.5842) -> (88.186, 208.9317) projected
  line L430 (88.186, 208.9317) -> (85.3218, 210.1176) projected
  line L431 (85.3218, 210.1176) -> (85.397, 212.3788) projected
  arc A143 (85.397, 212.3788) -> (80.9522, 214.1125) centre (0, 0) ccw projected
  line L432 (80.9522, 214.1125) -> (79.4766, 212.3975) projected
  line L433 (79.4766, 212.3975) -> (76.5658, 213.464) projected
  line L434 (76.5658, 213.464) -> (76.5475, 215.7264) projected
  arc A144 (76.5475, 215.7264) -> (72.0349, 217.2749) centre (0, 0) ccw projected
  line L435 (72.0349, 217.2749) -> (70.6313, 215.5004) projected
  line L436 (70.6313, 215.5004) -> (67.679, 216.4458) projected
  line L437 (67.679, 216.4458) -> (67.5672, 218.7055) projected
  arc A145 (67.5672, 218.7055) -> (62.9945, 220.0661) centre (0, 0) ccw projected
  line L438 (62.9945, 220.0661) -> (61.6655, 218.2352) projected
  line L439 (61.6655, 218.2352) -> (58.6766, 219.0577) projected
  line L440 (58.6766, 219.0577) -> (58.4715, 221.3108) projected
  arc A146 (58.4715, 221.3108) -> (53.8464, 222.4814) centre (0, 0) ccw projected
  line L441 (53.8464, 222.4814) -> (52.5942, 220.5971) projected
  line L442 (52.5942, 220.5971) -> (49.5739, 221.2954) projected
  line L443 (49.5739, 221.2954) -> (49.2759, 223.5381) projected
  arc A147 (49.2759, 223.5381) -> (44.6064, 224.5165) centre (0, 0) ccw projected
  line L444 (44.6064, 224.5165) -> (43.4331, 222.5821) projected
  line L445 (43.4331, 222.5821) -> (40.3865, 223.155) projected
  line L446 (40.3865, 223.155) -> (39.9961, 225.3835) projected
  arc A148 (39.9961, 225.3835) -> (35.2902, 226.1681) centre (0, 0) ccw projected
  line L447 (35.2902, 226.1681) -> (34.1978, 224.1868) projected
  line L448 (34.1978, 224.1868) -> (31.1302, 224.6333) projected
  line L449 (31.1302, 224.6333) -> (30.648, 226.8438) projected
  arc A149 (30.648, 226.8438) -> (25.9136, 227.4333) centre (0, 0) ccw projected
  line L450 (25.9136, 227.4333) -> (24.9041, 225.4085) projected
  line L451 (24.9041, 225.4085) -> (21.8206, 225.7279) projected
  line L452 (21.8206, 225.7279) -> (21.2475, 227.9165) projected
  arc A150 (21.2475, 227.9165) -> (16.4928, 228.3099) centre (0, 0) ccw projected
  circle A151 centre (0, 0) radius 236.22
  constraints: 1 centre point, 1 coincident
extrude "Extrusion14" add sketch "Sketch18" against normal blind 2.54 bodies 2
chamfer "Chamfer3" distance 1.27 angle 45 2 edges at (-236.22, 0, -2.54) (236.22, 0, -22.86)
sketch "Sketch25" plane through (0, 0, 0) normal (0, 0, 1) x (1, 0, 0)
  line L0 (-238.508, 0) -> (258.7625, 0)
  line L1 (258.7625, 0) -> (258.7625, 247.65)
  line L2 (258.7625, 247.65) -> (-238.508, 247.65)
  line L3 (-238.508, 247.65) -> (-238.508, 0)
  point P0 (0, 0)
  constraints: 8 end point, 2 parallel, 1 horizontal, 1 perpendicular
extrude "Extrusion19" cut sketch "Sketch25" against normal through all bodies 2
sketch "Sketch27" plane through (0, 0, -25.4) normal (0, 0, -1) x (-1, 0, 0)
  line L0 (63.5, 0) -> (236.22, 0) projected
  line L1 (223.52, 0) -> (160.02, 0)
  line L2 (160.02, 0) -> (160.02, -19.05)
  line L3 (160.02, -19.05) -> (223.52, -19.05)
  line L4 (223.52, -19.05) -> (223.52, 0)
  arc A0 (-98.1276, -19.05) -> (98.1276, -19.05) centre (0, 0) ccw projected
  line L5 (127, -19.05) -> (98.1276, -19.05) projected
  line L6 (-98.1276, -19.05) -> (-127, -19.05) projected
  line L7 (127, 0) -> (127, -19.05) projected
  line L8 (-127, -19.05) -> (-127, 0) projected
  arc A1 (-98.1276, -19.05) -> (98.1276, -19.05) centre (0, 0) ccw projected
  line L9 (0, -99.9596) -> (0, 0)
  line L10 (-223.52, 0) -> (-160.02, 0)
  line L11 (-160.02, 0) -> (-160.02, -19.05)
  line L12 (-160.02, -19.05) -> (-223.52, -19.05)
  line L13 (-223.52, -19.05) -> (-223.52, 0)
  dimension "d140" = 19.05
  dimension "d141" = 19.05
  dimension "d142" = 63.5
  dimension "d143" = 12.7
  constraints: 18 end point, 4 symmetric about line, 2 parallel, 2 point on circle, 1 horizontal, 1 perpendicular, 1 point on line, 1 vertical
  measures "d140" distance between parallel lines of L0 L5
  measures "d141" distance of L1.end L2.end
  measures "d142" distance of L2.end L3.end
  measures "d143" distance from line of L0.end L4
extrude "Extrusion20" add sketch "Sketch27" along normal blind 25.4 bodies 2
sketch "Sketch28" plane through (-223.52, -19.05, -25.4) normal (0, -1, 0) x (1, 0, 0)
  circle A0 centre (431.8, -12.7) radius 3.3782
  circle A1 centre (398.78, -12.7) radius 3.3782
  line L0 (447.04, 0) -> (447.04, -25.4) projected
  line L1 (383.54, 0) -> (383.54, -25.4) projected
  line L2 (447.04, -25.4) -> (383.54, -25.4) projected
  line L3 (321.6476, 50.8) -> (125.3924, 50.8) projected
  line L4 (223.52, 50.8) -> (223.52, -50.8)
  circle A2 centre (15.24, -12.7) radius 3.3782
  circle A3 centre (48.26, -12.7) radius 3.3782
  line L5 (0, 0) -> (0, -25.4)
  line L6 (63.5, 0) -> (63.5, -25.4)
  line L7 (0, -25.4) -> (63.5, -25.4)
  point P0 (223.52, 25.4)
  dimension "d146" = 6.7564
  dimension "d147" = 6.7564
  dimension "d148" = 15.24
  dimension "d149" = 15.24
  dimension "d150" = 12.7
  dimension "d151" = 25.4
  dimension "d152" = 12.7
  constraints: 8 end point, 6 symmetric about line, 4 centre point, 1 midpoint, 1 vertical, 2 other
  measures "d146" diameter of A0
  measures "d147" diameter of A1
  measures "d148" distance from line of L0 A0.centre
  measures "d149" distance from line of L1 A1.centre
  measures "d150" distance from line of L2 A1.centre
  measures "d151" distance of L1.start L1.end
  measures "d152" distance from line of L2 A0.centre
extrude "Extrusion21" cut sketch "Sketch28" against normal through all bodies 2
sketch "Sketch29" plane through (0, 0, -25.4) normal (0, 0, -1) x (-1, 0, 0)
  line L0 (0, 0) -> (0, -404.1913)
  line L1 (10.16, -139.7) -> (-10.16, -139.7)
  line L2 (63.5, -63.5) -> (-63.5, -63.5) projected
  arc A0 (-236.22, 0) -> (236.22, 0) centre (0, 0) ccw projected
  arc A1 (-10.16, -236.0014) -> (10.16, -236.0014) centre (0, 0) ccw
  line L3 (10.16, -236.0014) -> (10.16, -139.7)
  line L4 (-10.16, -139.7) -> (-10.16, -236.0014)
  dimension "d158" = 76.2
  dimension "d162" = 20.32
  dimension "d163" = 10.16
  dimension "d164" = 10.16
  constraints: 8 end point, 4 point on circle, 2 vertical, 1 centre point, 1 coincident, 1 horizontal, 1 parallel
  measures "d158" distance between parallel lines of L2 L1
  measures "d162" distance between parallel lines of L4 L3
  measures "d163" distance between parallel lines of L4 L0
  measures "d164" distance between parallel lines of L0 L3
extrude "Extrusion22" add sketch "Sketch29" along normal blind 20.32 bodies 2
sketch "Sketch32" plane through (0, 0, 0) normal (0, 0, 1) x (1, 0, 0)
  line L0 (10.16, -236.0014) -> (10.16, -139.7) projected
  line L1 (-10.16, -139.7) -> (-10.16, -236.0014) projected
  line L2 (10.16, -139.7) -> (-10.16, -139.7) projected
  arc A0 (-10.16, -236.0014) -> (10.16, -236.0014) centre (0, 0) ccw
  point P0 (0, 0)
  constraints: 2 point on circle, 1 centre point
extrude "Extrusion23" add sketch "Sketch32" along normal blind 20.32 bodies 2
sketch "Sketch33" plane through (-10.16, -236.0014, -25.4) normal (-1, 0, 0) x (0, 0, 1)
  circle A0 centre (-10.16, 24.0754) radius 3.3782
  circle A1 centre (-10.16, 48.1507) radius 3.3782
  circle A2 centre (-10.16, 72.2261) radius 3.3782
  line L0 (-20.32, 0) -> (-20.32, 96.3014) projected
  line L1 (0, 0) -> (0, 236.0014) projected
  line L2 (0, 96.3014) -> (-20.32, 96.3014) projected
  line L3 (0, 0) -> (-20.32, 0) projected
  circle A3 centre (35.56, 24.0754) radius 3.3782
  circle A4 centre (35.56, 48.1507) radius 3.3782
  circle A5 centre (35.56, 72.2261) radius 3.3782
  line L4 (45.72, 96.3014) -> (45.72, 0) projected
  point P0 (25.4, 236.0014)
  dimension "d167" = 6.7564
  dimension "d168" = 6.7564
  dimension "d169" = 6.7564
  dimension "d170" = 20.32
  dimension "d171" = 10.16
  dimension "d172" = 0
  dimension "d173" = 0
  dimension "d174" = 24.0754
  dimension "d175" = 96.3014
  dimension "d176" = 24.0754
  dimension "d177" = 24.0754
  dimension "d178" = 6.7564
  dimension "d179" = 6.7564
  dimension "d180" = 6.7564
  dimension "d181" = 0
  dimension "d182" = 0
  dimension "d183" = 24.0754
  dimension "d184" = 24.0754
  dimension "d187" = 10.16
  constraints: 6 centre point
  measures "d167" diameter of A0
  measures "d168" diameter of A1
  measures "d169" diameter of A2
  measures "d170" distance between parallel lines of L0 L1
  measures "d171" distance from line of L0 A0.centre
  measures "d172" horizontal distance of A0.centre A1.centre
  measures "d173" horizontal distance of A2.centre A1.centre
  measures "d174" distance from line of L2 A2.centre
  measures "d175" distance between parallel lines of L2 L3
  measures "d176" distance of A2.centre A1.centre
  measures "d177" distance of A1.centre A0.centre
  measures "d178" diameter of A3
  measures "d179" diameter of A4
  measures "d180" diameter of A5
  measures "d181" horizontal distance of A3.centre A4.centre
  measures "d182" horizontal distance of A5.centre A4.centre
  measures "d183" distance of A5.centre A4.centre
  measures "d184" distance of A4.centre A3.centre
  measures "d187" distance from line of L4 A3.centre
extrude "Extrusion24" cut sketch "Sketch33" against normal through all contours A0 | A1 | A2 | A3 | A4 | A5 bodies 2
sketch "Sketch35" plane through (0, 0, 25.4) normal (0, 0, 1) x (1, 0, 0)
  line L0 (45, -104.14) -> (-45, -104.14)
  line L1 (45, -104.14) -> (45, -89.2577)
  arc A0 (-98.1276, -19.05) -> (98.1276, -19.05) centre (0, 0) ccw projected
  line L2 (-45, -104.14) -> (-45, -89.2577)
  arc A1 (-45, -89.2577) -> (45, -89.2577) centre (0, 0) ccw
  dimension "d195" = 104.14
  dimension "d196" = 90
  constraints: 6 end point, 4 point on circle, 1 centre point, 1 coincident, 1 horizontal, 1 parallel, 1 vertical
  measures "d195" distance from line of point (0, 0) L0
  measures "d196" distance of L0.start L0.end
extrude "Extrusion26" add sketch "Sketch35" against normal up to surface (25.4 mm away) bodies 1
sketch "Sketch36" plane through (-45, -104.14, 25.4) normal (0, -1, 0) x (1, 0, 0)
  circle A0 centre (76.5, -12.7) radius 4
  circle A1 centre (13.5, -12.7) radius 4
  line L0 (90, 0) -> (90, -25.4) projected
  line L1 (0, 0) -> (90, 0) projected
  line L2 (0, 0) -> (0, -25.4) projected
  point P0 (45, -25.4)
  dimension "d200" = 63
  dimension "d201" = 8
  dimension "d202" = 8
  dimension "d203" = 13.5
  dimension "d204" = 12.7
  dimension "d205" = 13.5
  dimension "d206" = 12.7
  constraints: 2 centre point
  measures "d200" distance of A1.centre A0.centre
  measures "d201" diameter of A0
  measures "d202" diameter of A1
  measures "d203" distance from line of A0.centre L0
  measures "d204" distance from line of L1 A0.centre
  measures "d205" distance from line of L2 A1.centre
  measures "d206" distance from line of L1 A1.centre
extrude "Extrusion27" cut sketch "Sketch36" against normal blind 10 bodies 1
sketch "Sketch37" plane through (0, 0, -25.4) normal (0, 0, -1) x (-1, 0, 0)
  line L0 (0, 0) -> (271.4625, 0)
  line L1 (271.4625, 0) -> (271.4625, -287.3375)
  line L2 (271.4625, -287.3375) -> (0, -287.3375)
  line L3 (0, -287.3375) -> (0, 0)
  constraints: 8 end point, 2 parallel, 1 horizontal, 1 perpendicular
extrude "Extrusion28" cut sketch "Sketch37" along normal mid plane 200 bodies 2
sketch "Sketch38" plane through (0, 0, 25.4) normal (0, 0, 1) x (1, 0, 0)
  line L0 (0, 0) -> (-185.7375, 0)
  line L1 (-185.7375, 0) -> (-185.7375, -146.05)
  line L2 (-185.7375, -146.05) -> (0, -146.05)
  line L3 (0, -146.05) -> (0, 0)
  constraints: 8 end point, 2 parallel, 1 horizontal, 1 perpendicular
extrude "Extrusion29" cut sketch "Sketch38" against normal blind 200 bodies 1
sketch "Sketch40" plane through (0, 0, -25.4) normal (0, 0, -1) x (-1, 0, 0)
  circle A0 centre (-185.42, -95.25) radius 5
  circle A1 centre (-185.42, -69.85) radius 5
  line L0 (-223.52, 0) -> (-223.52, -19.05) projected
  line L1 (-160.02, -19.05) -> (-223.52, -19.05) projected
  point P0 (0, 0)
  dimension "d213" = 10
  dimension "d214" = 38.1
  dimension "d215" = 25.4
  dimension "d216" = 0
  dimension "d217" = 50.8
  dimension "d218" = 10
  constraints: 2 centre point
  measures "d213" diameter of A0
  measures "d214" distance from line of L0 A0.centre
  measures "d215" distance of A0.centre A1.centre
  measures "d216" horizontal distance of A1.centre A0.centre
  measures "d217" distance from line of L1 A1.centre
  measures "d218" diameter of A1
extrude "Extrusion30" cut sketch "Sketch40" against normal through all bodies 2
fillet "Fillet3" radius 1.27 4 edges at (190.42, -95.25, -25.4) (190.42, -69.85, -25.4) (190.42, -95.25, 0) (190.42, -69.85, 0)
equation "\"d36\" = 0.25 * d33"
equation "\"d39\" = 0.25 * d33"
equation "\"d41\" = d40"
equation "\"d37\" = d36"
body "Solid1"
body "Solid3"
